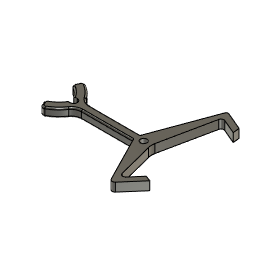
PalletFork v5 (Autodesk Fusion 360 design; units mm, degrees)
Autodesk Fusion 360 part; units mm, degrees
sketch "main" plane through (0, 0, 0) normal (0, 0, 1) x (1, 0, 0)
  circle A0 centre (21.8365, 0.0332) radius 2.25
  line L0 (-29.4135, 2.5332) -> (-26.9135, 2.5332)
  line L1 (-26.9135, -2.4668) -> (-29.4135, -2.4668)
  line L2 (-34.9258, 10.2857) -> (-33.9469, 12.3465) construction
  line L3 (-35.7535, 13.2046) -> (-36.7324, 11.1438)
  arc A1 (-32.9614, 14.0869) -> (-35.7535, 13.2046) centre (-33.9469, 12.3465) ccw
  arc A2 (-36.7324, 11.1438) -> (-35.9243, 8.5528) centre (-34.9258, 10.2857) ccw
  arc A3 (-24.2048, 6.0328) -> (-32.9614, 14.0869) centre (-45.9085, -8.7768) ccw
  line L4 (-36.7417, -11.0419) -> (-35.7592, -13.1001)
  arc A4 (-35.9295, -8.4441) -> (-36.7417, -11.0419) centre (-34.9367, -10.1804) ccw
  arc A5 (-35.7592, -13.1001) -> (-32.8186, -13.8848) centre (-33.9543, -12.2386) ccw
  line L5 (-32.8186, -13.8848) -> (-32.8147, -13.8915) construction
  arc A6 (-35.9295, -8.4441) -> (-29.4135, -2.4668) centre (-45.8569, 8.9181) ccw
  arc A7 (-26.9362, -2.4667) -> (-26.9135, 2.5332) centre (-26.9135, 0.0332) ccw
  arc A8 (-29.4135, 2.5332) -> (-35.9243, 8.5528) centre (-45.9085, -8.7768) ccw
  arc A9 (-26.9361, -2.4668) -> (-26.9362, -2.4667) centre (-45.9085, -8.7768) ccw
  arc A10 (-32.9737, -13.9817) -> (-24.2534, -6.0374) centre (-45.8569, 8.9181) ccw
  circle A11 centre (-18.4227, 9.9783) radius 7
  circle A12 centre (-18.498, -10.0217) radius 7
  line L6 (-18.4227, 2.9783) -> (17.5773, 2.9783)
  line L7 (-18.498, -3.0217) -> (17.502, -3.0217)
  line L8 (17.5773, 2.9783) -> (33.1079, 45.2119)
  line L9 (17.502, -3.0217) -> (33.4968, -34.2782)
  line L10 (47.9397, -21.8492) -> (36.7867, -34.6793)
  arc A13 (33.4968, -34.2782) -> (36.7867, -34.6793) centre (35.2773, -33.3672) ccw
  line L11 (47.9397, -21.8492) -> (43.9626, -20.3226)
  line L12 (43.9626, -20.3226) -> (37.3696, -27.907)
  line L13 (27.4111, -2.1643) -> (33.9251, -27.1004)
  arc A14 (33.9251, -27.1004) -> (37.3696, -27.907) centre (35.8602, -26.5949) ccw
  line L14 (27.2967, 2.403) -> (34.9624, 39.1928)
  arc A15 (27.2967, 2.403) -> (27.4111, -2.1643) centre (37.0865, 0.3632) ccw
  line L15 (37.7018, 40.6259) -> (47.9839, 36.2614)
  arc A16 (37.7018, 40.6259) -> (34.9624, 39.1928) centre (36.9204, 38.7849) ccw
  line L16 (47.9839, 36.2614) -> (47.421, 40.8458)
  line L17 (35.1018, 46.075) -> (47.421, 40.8458)
  arc A17 (35.1018, 46.075) -> (33.1079, 45.2119) centre (34.5157, 44.6942) ccw
  dimension "d1" = 5
  dimension "d3" = 4.5
  dimension "d4" = 2.5
  dimension "d5" = 40
  dimension "d6" = 40
  dimension "d7" = 4
  dimension "d9" = 4
  dimension "d11" = 52.55
  dimension "d12" = 52.55
  dimension "d13" = 4
  dimension "d14" = 4
  dimension "d15" = 14
  dimension "d16" = 14
  dimension "d17" = 20
  dimension "d20" = 110.19
  dimension "d22" = 117.1
  dimension "d25" = 68.1
  dimension "d26" = 2
  dimension "d27" = 17
  dimension "d28" = 4.26
  dimension "d29" = 70
  dimension "d30" = 110
  dimension "d31" = 55.64
  dimension "d32" = 2
  dimension "d33" = 153.59
  dimension "d34" = 10
  dimension "d35" = 78.77
  dimension "d36" = 2
  dimension "d37" = 11.17
  dimension "d38" = 60
  dimension "d39" = 120
  dimension "d40" = 4
  dimension "d41" = 1.5
  dimension "d45" = 48.75
  dimension "d47" = 15.25
  dimension "d48" = 36
  dimension "d49" = 6
  constraint horizontal L0
  constraint tangent L0 A7
  constraint horizontal L1
  constraint tangent L1 A7
  constraint coincident L1.start A7
  constraint equal L0 L1
  constraint tangent A2 A8
  constraint coincident L2.start A2.centre
  constraint coincident L2.end A1.centre
  constraint parallel L2 L3
  constraint tangent L3 A2
  constraint concentric A3 A8
  constraint tangent A1 A3
  constraint concentric A6 A10
  constraint tangent A4 A6
  constraint tangent A5 A10
  constraint tangent L4 A4
  constraint tangent L4 A5
  constraint coincident L5.end A10
  constraint coincident L1 A9.start
  constraint concentric A8 A9
  constraint coincident A5 A10.start
  constraint tangent A3 A11
  constraint tangent A10 A12
  constraint tangent A11 L6
  constraint coincident A11 L6.start
  constraint horizontal L7
  constraint tangent A12 L7
  constraint coincident A12 L7.start
  constraint tangent L9 A13
  constraint tangent L10 A13
  constraint tangent L13 A14
  constraint tangent L12 A14
  constraint tangent L14 A15
  constraint tangent L13 A15
  constraint tangent L14 A16
  constraint tangent L15 A16
  constraint coincident L15.end L16.start
  constraint tangent L8 A17
  constraint tangent L17 A17
  constraint coincident A11 A3.start
  constraint coincident A12 A10.end
  constraint horizontal A7.centre A0.centre
  constraint equal L6 L7
  measures "d1" diameter of A7
  measures "d3" diameter of A0
  measures "d4" distance of L0.start L0.end
  measures "d5" diameter of A8
  measures "d6" diameter of A6
  measures "d7" diameter of A2
  measures "d9" diameter of A1
  measures "d11" diameter of A3
  measures "d12" diameter of A10
  measures "d13" diameter of A4
  measures "d14" diameter of A5
  measures "d15" diameter of A11
  measures "d16" diameter of A12
  measures "d17" vertical distance of A11.centre A12.centre
  measures "d20" angle of L6 L8
  measures "d22" angle of L7 L9
  measures "d25" angle of L9 L10
  measures "d26" radius of A13
  measures "d27" distance of L10.start L10.end
  measures "d28" distance of L10.start L11.end
  measures "d29" angle of L10 L11
  measures "d30" angle of L11 L12
  measures "d31" angle of L12 L13
  measures "d32" radius of A14
  measures "d33" angle of L13 L14
  measures "d34" radius of A15
  measures "d35" angle of L14 L15
  measures "d36" radius of A16
  measures "d37" distance of L15.end L15.start
  measures "d38" angle of L15 L16
  measures "d39" angle of L16 L17
  measures "d40" distance of L15 L17
  measures "d41" radius of A17
  measures "d45" horizontal distance of A7.centre A0.centre
  measures "d47" horizontal distance of A0.centre A15.centre
  measures "d48" distance of L6.end L6.start
  measures "d49" vertical distance of L6.end L7.end
extrude "Extrude1" add sketch "main" along normal blind 6 contours L0 L1 L3 A1 A2 A3 A7 A8 A9 A10 A11 A12 L6 L7 L8 L9 L10 A13 L11 L12 L13 A14 L14 A15 L15 A16 L16 L17 A17 | L1 L4 A4 A5 A6 A9 A10 picked at (-28.4657, -7.1435)
fillet "Fillet1" radius 1 28 edges at (-0.4227, 2.9783, 6) (-21.6924, 3.7889, 6) (-28.1213, 10.562, 6) (-34.5495, 14.2536, 6) (-36.2429, 12.1742, 6) (-36.8351, 9.6902, 6) (-32.3311, 5.9083, 6) (-32.337, -5.8201, 6) (-36.8456, -9.5835, 6) (-36.2504, -12.071, 6) (-34.5578, -14.1454, 6) (-28.1619, -10.5052, 6) (-21.7468, -3.8213, 6) (-0.498, -3.0217, 6) (-32.337, -5.8201, 0) (-36.8456, -9.5835, 0) (-36.2504, -12.071, 0) (-34.5578, -14.1454, 0) (-28.1619, -10.5052, 0) (-21.7468, -3.8213, 0) (-0.498, -3.0217, 0) (-0.4227, 2.9783, 0) (-21.6924, 3.7889, 0) (-28.1213, 10.562, 0) (-34.5495, 14.2536, 0) (-36.2429, 12.1742, 0) (-36.8351, 9.6902, 0) (-32.3311, 5.9083, 0)
equation "d47 = 13 mm + 2.25 mm"
named bodies: "PalletFork"
